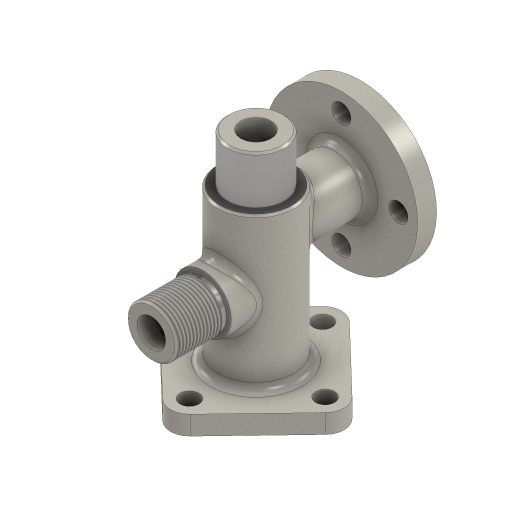
# Autodesk Inventor part: Part035.Valve Body
Saved by Autodesk Inventor 2023.2 (Build 272271030, 271C)
## iProperties
Created: 2023-11-15
Part Number: Part035.Valve Body
Material: Steel, Carbon
Document SubType Name: Modeling
Designer: User
Mass: 1427.74 g
Surface Area: 535.64 cm^2
Volume: 181.878 cm^3
Density: 7.85 g/cm^3
Appearance: Steel - Cast
Author: User
Autodesk Inventor part; units mm, degrees
ref_plane "YZ Plane" through (0, 0, 0) normal (1, 0, 0) x (0, 1, 0)
ref_plane "XZ Plane" through (0, 0, 0) normal (0, 1, 0) x (-1, 0, 0)
ref_plane "XY Plane" through (0, 0, 0) normal (0, 0, 1) x (1, 0, 0)
sketch "Sketch1" plane through (0, 0, 0) normal (0, 1, 0) x (-1, 0, 0)
  line L0 (0, 35) -> (33.5289, 2.7993) construction
  line L1 (33.5861, -0.0286) -> (0, -35) construction
  line L2 (0, -35) -> (-34.9714, -1.4139) construction
  line L3 (-34.9714, -1.4139) -> (0, 35) construction
  line L4 (0, 35) -> (0, -35) construction
  line L5 (34.9714, 1.4139) -> (-34.9714, -1.4139) construction
  line L6 (7.2125, -41.9268) -> (42.1839, -5.5128)
  line L7 (41.8982, 8.6264) -> (6.9268, 42.2125)
  line L8 (-7.2125, 41.9268) -> (-42.1839, 5.5128)
  line L9 (-41.8982, -8.6264) -> (-6.9268, -42.2125)
  arc A0 (33.5861, -0.0286) -> (33.5289, 2.7993) centre (32.1436, 1.3568) ccw
  arc A1 (-6.9268, -42.2125) -> (7.2125, -41.9268) centre (0, -35) ccw
  arc A2 (-42.1839, 5.5128) -> (-41.8982, -8.6264) centre (-34.9714, -1.4139) ccw
  arc A3 (42.1839, -5.5128) -> (41.8982, 8.6264) centre (34.9714, 1.4139) ccw
  arc A4 (6.9268, 42.2125) -> (-7.2125, 41.9268) centre (0, 35) ccw
  point P0 (0, 0)
  dimension "d0" = 70
  dimension "d1" = 10
  dimension "d2" = 2
  dimension "d3" = 10
  constraints: 20 end point, 10 point on circle, 10 tangent, 5 centre point, 4 parallel, 3 equal radius, 3 perpendicular, 2 midpoint, 2 point on line, 1 vertical, 3 other
  measures "d0" distance of L0.start L1.end
  measures "d1" distance between parallel lines of L1 L6
  measures "d2" radius of A0
  measures "d3" radius of A1
extrude "Extrusion1" add sketch "Sketch1" along normal blind 10
sketch "Sketch2" plane through (0, 0, 0) normal (0, 0, 1) x (1, 0, 0)
  line L0 (-20, 10) -> (-20, 90)
  line L1 (-20, 90) -> (-15, 90)
  line L2 (-15, 90) -> (-15, 115)
  line L3 (-15, 115) -> (0, 115)
  line L4 (0, 115) -> (0, 10)
  line L5 (0, 10) -> (-20, 10)
  line L6 (-7.2125, 10) -> (-42.1839, 10) projected
  point P0 (0, 0)
  dimension "d7" = 30
  dimension "d8" = 115
  dimension "d9" = 40
  dimension "d10" = 25
  constraints: 12 end point, 4 perpendicular, 2 vertical, 1 collinear, 1 point on line
  measures "d7" diameter of L2 L4
  measures "d8" distance from line of point (0, 0) L3
  measures "d9" diameter of L0 L4
  measures "d10" distance of L1.end L2.end
revolve "Revolution1" add sketch "Sketch2" angle 360 about axis through (0, 115, 0) along (0, -1, 0)
sketch "Sketch3" plane through (0, 0, 0) normal (1, 0, 0) x (0, 1, 0)
  line L0 (50, 0) -> (50, 55)
  line L1 (50, 55) -> (63.2205, 55)
  line L2 (63.2205, 55) -> (63.2205, 31)
  line L3 (63.2205, 31) -> (62.5, 31)
  line L4 (62.5, 31) -> (62.5, 28)
  line L5 (62.5, 28) -> (65, 28)
  line L6 (65, 28) -> (65, 0)
  line L7 (65, 0) -> (50, 0)
  point P0 (0, 0)
  dimension "d12" = 26.441
  dimension "d13" = 25
  dimension "d16" = 30
  dimension "d17" = 55
  dimension "d18" = 27
  dimension "d19" = 3
  dimension "d20" = 50
  constraints: 16 end point, 5 perpendicular, 2 horizontal, 1 point on line, 1 vertical
  measures "d12" diameter of L2 L0
  measures "d13" diameter of L4 L0
  measures "d16" diameter of L6 L0
  measures "d17" distance between parallel lines of L1 L7
  measures "d18" distance between parallel lines of L1 L5
  measures "d19" distance between parallel lines of L5 L3
  measures "d20" distance from line of point (0, 0) L0
revolve "Revolution2" add sketch "Sketch3" angle 360 about axis through (0, 50, 0) along (0, 0, 1)
sketch "Sketch4" plane through (0, 0, 0) normal (1, 0, 0) x (0, 1, 0)
  line L0 (70, 0) -> (70, -55)
  line L1 (70, -55) -> (110, -55)
  line L2 (110, -55) -> (110, -45)
  line L3 (110, -45) -> (85, -45)
  line L4 (85, -45) -> (85, 0)
  line L5 (85, 0) -> (70, 0)
  line L6 (63.2205, 55) -> (36.7795, 55) projected
  point P0 (0, 0)
  dimension "d22" = 80
  dimension "d23" = 10
  dimension "d24" = 30
  dimension "d25" = 110
  dimension "d26" = 70
  constraints: 12 end point, 3 perpendicular, 2 horizontal, 1 point on line, 1 vertical
  measures "d22" diameter of L2 L0
  measures "d23" distance between parallel lines of L1 L3
  measures "d24" diameter of L4 L0
  measures "d25" distance between parallel lines of L6 L1
  measures "d26" distance from line of point (0, 0) L0
revolve "Revolution3" add sketch "Sketch4" angle 360 about axis through (0, 70, 0) along (0, 0, -1)
sketch "Sketch5" plane through (0, 0, 0) normal (1, 0, 0) x (0, 1, 0)
  line L0 (115, 15) -> (115, -15) projected
  line L1 (115, 0) -> (0, 0)
  line L2 (0, 0) -> (0, 15)
  line L3 (0, -5.5128) -> (0, 8.6264) projected
  line L4 (0, 15) -> (35, 12.5)
  line L5 (35, 12.5) -> (85, 12.5)
  line L6 (85, 12.5) -> (85, 8)
  line L7 (85, 8) -> (115, 8)
  line L8 (115, 8) -> (115, 0)
  dimension "d28" = 25
  dimension "d29" = 30
  dimension "d30" = 35
  dimension "d31" = 16
  dimension "d32" = 30
  constraints: 14 end point, 3 perpendicular, 1 collinear, 1 horizontal, 1 midpoint, 1 parallel
  measures "d28" diameter of L5 L1
  measures "d29" diameter of L2.end L1
  measures "d30" horizontal distance of L1.end L4.end
  measures "d31" diameter of L7 L1
  measures "d32" distance between parallel lines of L0 L6
revolve "Revolution4" cut sketch "Sketch5" angle 360 about axis through (0, 115, 0) along (0, -1, 0)
sketch "Sketch6" plane through (0, 50, 55) normal (0, 0, 1) x (1, 0, 0)
  circle A0 centre (0, 0) radius 13.2205 projected
  circle A1 centre (0, 0) radius 7.5
  point P0 (0, -50)
  dimension "d34" = 15
  constraints: 1 centre point, 1 coincident
  measures "d34" diameter of A1
extrude "Extrusion2" cut sketch "Sketch6" against normal up to surface contours A1
sketch "Sketch7" plane through (0, 0, 0) normal (1, 0, 0) x (0, 1, 0)
  line L0 (70, 0) -> (70, -55)
  line L1 (30, -55) -> (110, -55) projected
  line L2 (70, -55) -> (90, -55)
  line L3 (90, -53) -> (77.5, -53)
  line L4 (77.5, -53) -> (77.5, 0)
  line L5 (77.5, 0) -> (70, 0)
  line L6 (90, -53) -> (90, -55)
  point P0 (0, 0)
  dimension "d37" = 2
  dimension "d38" = 40
  dimension "d39" = 15
  constraints: 12 end point, 2 perpendicular, 2 vertical, 1 horizontal, 1 midpoint, 1 point on line
  measures "d37" distance between parallel lines of L1 L3
  measures "d38" diameter of L6 L0
  measures "d39" diameter of L4 L0
revolve "Revolution5" cut sketch "Sketch7" angle 360 about axis through (0, 70, 0) along (0, 0, -1)
thread "Thread1" size "G 3/4-14" class "A" standard "BSP Pipe Threads" full length
chamfer "Chamfer1" distance 1 angle 45 3 edges at (15, 115, 0) (20, 90, 0) (0, 36.7795, 55)
fillet "Fillet1" radius 4 4 edges at (0, 55, -45) (0.0643, 35.0001, 19.9999) (-0.0643, 55.0001, -19.9999) (20, 10, 0)
sketch "Sketch8" plane through (0, 0, 0) normal (0, -1, 0) x (1, 0, 0)
  arc A0 (-41.8982, 8.6264) -> (-42.1839, -5.5128) centre (-34.9714, 1.4139) ccw projected
  arc A1 (-7.2125, -41.9268) -> (6.9268, -42.2125) centre (0, -35) ccw projected
  arc A2 (41.8982, -8.6264) -> (42.1839, 5.5128) centre (34.9714, -1.4139) ccw projected
  arc A3 (7.2125, 41.9268) -> (-6.9268, 42.2125) centre (0, 35) ccw projected
hole "Hole1" at (34.9714, 0, -1.4139) at (0, 0, 35) at (0, 0, -35) at (-34.9714, 0, 1.4139) direction (0, 1, 0) diameter 10 depth 10
sketch "Sketch9" plane through (0, 70, -55) normal (0, 0, -1) x (-1, 0, 0)
  circle A0 centre (0, 0) radius 20 projected
  line L0 (-18.8674, 28.6647) -> (21.3831, 28.6647)
  point P0 (0, -70)
  point P1 (0, 30)
  dimension "d54" = 30
  constraints: 2 end point, 1 horizontal, 1 vertical alignment
  measures "d54" distance of A0.centre point (0, 30)
hole "Hole2" at (0, 100, -55) direction (0, 0, 1) diameter 10 depth 10
pattern_circular "Circular Pattern1" count 4 over 360 about axis through (0, 70, -50) along (0, 0, -1) of "Hole2"
body "Solid1"
